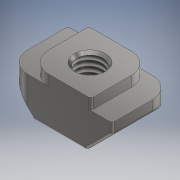
# Autodesk Inventor part: Noix M3
Saved by Autodesk Inventor 2017 (Build 210142000, 142)
## iProperties
Company: FABLAB Frenchmakers
Part Number: Noix M3
Material: Acier inoxydable
Document SubType Name: Modeling
Designer: FABLAB Frenchmakers
Density: 8 g/cm^3
Appearance: Semi-poli
Mass: 1.40079 g
Surface Area: 2.33869 cm^2
Volume: 0.175099 cm^3
Stock Number: 1420-01-11
Project: 1420 Vauban 3D XL
Catalog Web Link: http://frenchmakers.com/
Autodesk Inventor part; units mm, degrees
ref_plane "YZ Plane" through (0, 0, 0) normal (1, 0, 0) x (0, 1, 0)
ref_plane "XZ Plane" through (0, 0, 0) normal (0, 1, 0) x (-1, 0, 0)
ref_plane "XY Plane" through (0, 0, 0) normal (0, 0, 1) x (1, 0, 0)
sketch "Esquisse1" plane through (0, 0, 0) normal (0, 0, 1) x (1, 0, 0)
  line L0 (-5, -2.9) -> (5, -2.9)
  line L1 (5, -2.9) -> (5, 2.9)
  line L2 (5, 2.9) -> (-5, 2.9)
  line L3 (-5, 2.9) -> (-5, -2.9)
  line L4 (-5, -2.9) -> (5, 2.9) construction
  line L5 (5, -2.9) -> (-5, 2.9) construction
  point P0 (0, 0)
  dimension "d0" = 10
  dimension "d1" = 5.8
  constraints: 12 end point, 2 midpoint, 2 parallel, 1 horizontal, 1 perpendicular
  measures "d0" distance between parallel lines of L1 L3
  measures "d1" distance between parallel lines of L0 L2
extrude "Extrusion1" add sketch "Esquisse1" along normal blind 3.5
chamfer "Chanfrein1" distance 2.5 angle 45 2 edges at (5, 0, 0) (-5, 0, 0)
fillet "Congé1" radius 2 2 edges at (5, 2.9, 3) (-5, -2.9, 3)
fillet "Congé2" radius 0.25 12 edges at (0, 2.9, 0) (5, -1, 2.5) (4.4142, 2.3142, 1.9142) (3.75, -2.9, 1.25) (0, -2.9, 0) (2.5, 0, 0) (-2.5, 0, 0) (-3.75, 2.9, 1.25) (-5, 1, 2.5) (-4.4142, -2.3142, 1.9142) (-5, 2.9, 3) (5, -2.9, 3)
sketch "Esquisse2" plane through (0, 0, 3.5) normal (0, 0, 1) x (1, 0, 0)
  line L0 (3, 2.9) -> (-3, 2.9)
  line L1 (-3, 2.9) -> (-3, -2.9)
  line L2 (-3, -2.9) -> (3, -2.9)
  line L3 (3, -2.9) -> (3, 2.9)
  line L4 (3, 2.9) -> (-3, -2.9) construction
  line L5 (-3, 2.9) -> (3, -2.9) construction
  line L6 (-3, -2.9) -> (4.75, -2.9) projected
  point P0 (0, 0)
  dimension "d9" = 6
  constraints: 12 end point, 2 midpoint, 2 parallel, 1 collinear, 1 horizontal, 1 perpendicular
  measures "d9" distance between parallel lines of L3 L1
extrude "Extrusion2" add sketch "Esquisse2" along normal blind 1
fillet "Congé3" radius 2 2 edges at (3, 2.9, 4) (-3, -2.9, 4)
fillet "Congé4" radius 0.25 2 edges at (-3, 2.9, 4) (3, -2.9, 4)
sketch "Esquisse3" plane through (0, 0, 4.5) normal (0, 0, 1) x (1, 0, 0)
  point P0 (0, 0)
  point P1 (0, 0)
  constraints: 1 coincident
hole "Perçage1" at (0, 0, 4.5) direction (0, 0, -1) diameter 2.459 depth 8.8 tip angle 118 thread size "M3x0.5" class "6H" standard "ISO Metric profile"
chamfer "Chanfrein2" distance 0.25 angle 45 2 edges at (0, 1.2295, 4.5) (0, 1.2295, 0)
